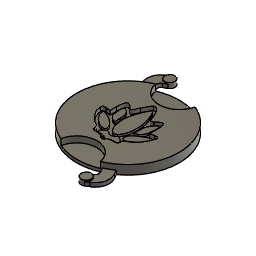
Deckbox - Key - Fungus (Autodesk Fusion 360 design; units mm, degrees)
Autodesk Fusion 360 part; units mm, degrees
sketch "Sketch1" plane through (0, 0, 0) normal (0, 1, 0) x (1, 0, 0)
  circle A0 centre (0, 0) radius 25.4
  line L0 (19.5918, -28.934) -> (-15.2617, 31.434)
  line L1 (-19.5918, 28.934) -> (15.2617, -31.434)
  line L2 (0, -25.4) -> (0, 25.4) construction
  line L3 (0, 0) -> (25.4, 0) construction
  line L4 (-19.5918, 28.934) -> (-15.2617, 31.434)
  line L5 (15.2617, -31.434) -> (19.5918, -28.934)
  line L6 (17.4268, -30.184) -> (-17.4268, 30.184) construction
  line L7 (-2.1651, -1.25) -> (2.1651, 1.25) construction
  line L8 (19.5918, -28.934) -> (11.7976, -33.434)
  line L9 (11.7976, -33.434) -> (9.2976, -29.1039)
  line L10 (9.2976, -29.1039) -> (17.0918, -24.6039)
  line L11 (17.0918, -24.6039) -> (19.5918, -28.934)
  circle A1 centre (10.5476, -31.269) radius 2.5
  circle A2 centre (0, 0) radius 35.5
  line L12 (-19.5918, 28.934) -> (-17.0918, 24.6039)
  line L13 (-17.0918, 24.6039) -> (-9.2976, 29.1039)
  line L14 (-9.2976, 29.1039) -> (-11.7976, 33.434)
  line L15 (-11.7976, 33.434) -> (-19.5918, 28.934)
  circle A3 centre (-10.5476, 31.269) radius 2.5
  point P0 (-12.5, 21.6506)
  point P1 (12.5, -21.6506)
  dimension "d1" = 50.8
  dimension "d42" = 5
  dimension "d45" = 5
  dimension "d46" = 71
  dimension "d47" = 60
  dimension "d48" = 4
  dimension "d51" = 5
  constraint coincident A0.centre L3.start
  constraint coincident A0 L2.start
  constraint coincident A0 L2.end
  constraint coincident A0.centre L2
  constraint coincident A0 L3.end
  constraint horizontal L3
  constraint perpendicular L0 L4
  constraint perpendicular L0 L5
  constraint perpendicular L1 L4
  constraint midpoint L5 L6.start
  constraint midpoint L4 L6.end
  constraint perpendicular L4 L6
  constraint midpoint L1 L7.start
  constraint midpoint L0 L7.end
  constraint midpoint L6 A0.centre
  constraint perpendicular L8 L9
  constraint parallel L8 L10
  constraint parallel L9 L11
  constraint perpendicular L0 L8
  constraint midpoint L9 A1.centre
  constraint tangent L10 A1
  constraint concentric A0 A2
  constraint tangent A1 A2
  constraint perpendicular L12 L13
  constraint parallel L12 L14
  constraint parallel L13 L15
  constraint coincident L1 L12.end
  constraint midpoint L14 A3.centre
  constraint tangent L13 A3
  constraint tangent A2 A3
  measures "d1" diameter of A0
  measures "d42" distance of L0 L1
  measures "d45" diameter of A1
  measures "d46" diameter of A2 A0.centre
  measures "d47" angle of L3 L6
  measures "d48" distance of L1 A1.centre
  measures "d51" diameter of A3
extrude "Extrude1" add sketch "Sketch1" along normal blind 4.5 contours A0 L0 | A0 L0 L1 | A0 L1
extrude "Extrude2" add sketch "Sketch1" along normal blind 1.9 contours A0 L0 | A0 L0 L1 | A0 L0 L1 L13 | A0 L0 L1 L10 | A0 L1 | L0 L1 L4 L12 L13 L15 | L0 L13 L15 A3 | L0 L1 L5 L8 L10 L11 | L14 A3 | L14 A3 | L1 L8 L10 A1 | L9 A1 | L9 A1
extrude "Extrude3" add sketch "Sketch1" along normal blind 2.5 contours L14 A3 | L14 A3 | L9 A1 | L9 A1
sketch "Sketch2" plane through (0, 4.5, 0) normal (0, 1, 0) x (-1, 0, 0)
  circle A0 centre (0, 0) radius 25.4
  circle A1 centre (0, -25.4) radius 10
  circle A2 centre (0, 25.4) radius 10
  line L0 (0, -25.4) -> (0, 25.4) construction
  dimension "d18" = 20
  dimension "d19" = 20
  constraint coincident A0 A1.centre
  constraint coincident A0 A2.centre
  constraint coincident A1.centre L0.start
  constraint coincident A2.centre L0.end
  constraint coincident A0.centre L0
  constraint vertical L0
  measures "d18" diameter of A1
  measures "d19" diameter of A2
extrude "Extrude4" cut sketch "Sketch2" against normal blind 3 contours A0 A2 | A0 A1 picked at (-1.832, 22.0709) picked at (1.832, -22.0709)
fillet "Fillet6" radius 2 2 edges at (12.7617, 0.95, 27.1039) (-12.7617, 0.95, -27.1039)
fillet "Fillet7" radius 7 2 edges at (19.5918, 0.95, 28.934) (-19.5918, 0.95, -28.934)
sketch "Sketch4" plane through (0, 4.5, 0) normal (0, 1, 0) x (-1, 0, 0)
  arc A0 (-9.8043, 23.4315) -> (9.8043, 23.4315) centre (0, 25.4) ccw
  arc A1 (-9.8043, 23.4315) -> (-9.8043, -23.4315) centre (0, 0) ccw
  arc A2 (9.8043, -23.4315) -> (-9.8043, -23.4315) centre (0, -25.4) ccw
  arc A3 (9.8043, -23.4315) -> (9.8043, 23.4315) centre (0, 0) ccw
  spline S0 degree 3 poles (0.8971, -13.3881) (1.2668, -13.1528) (2.3293, -11.3261) (3.2581, -9.3287) knots 0 0 0 0 1 1 1 1
  spline S1 degree 3 poles (3.2581, -9.3287) (4.7374, -6.1473) (5.0418, -5.8117) (5.7137, -6.6214) knots 0 0 0 0 1 1 1 1
  spline S2 degree 3 poles (5.7137, -6.6214) (8.3263, -9.7693) (9.7289, -8.853) (9.7424, -3.9899) knots 0 0 0 0 1 1 1 1
  line L0 (9.7424, -3.9899) -> (9.7512, -0.786)
  line L1 (9.7512, -0.786) -> (11.8532, -1.0314)
  spline S3 degree 3 poles (11.8532, -1.0314) (13.8107, -1.2599) (13.6243, -0.8636) (13.5174, 0.1243) knots 0 0 0 0 1 1 1 1
  spline S4 degree 3 poles (13.5174, 0.1243) (13.3689, 2.9805) (12.268, 3.8405) (11.0374, 5.5764) knots 0 0 0 0 1 1 1 1
  spline S5 degree 3 poles (11.0374, 5.5764) (10.3465, 6.5665) (8.995, 7.7022) (8.0341, 8.1002) knots 0 0 0 0 1 1 1 1
  spline S6 degree 3 poles (8.0341, 8.1002) (6.782, 8.6189) (6.287, 9.213) (6.287, 10.1973) knots 0 0 0 0 1 1 1 1
  spline S7 degree 3 poles (6.287, 10.1973) (6.287, 11.4074) (6.0209, 11.5706) (4.0482, 11.5706) knots 0 0 0 0 1 1 1 1
  spline S8 degree 3 poles (4.0482, 11.5706) (2.7625, 11.5706) (1.5034, 11.9394) (1.0907, 12.4367) knots 0 0 0 0 1 1 1 1
  spline S9 degree 3 poles (1.0907, 12.4367) (0.17, 13.546) (-1.0019, 13.546) (-1.4276, 12.4367) knots 0 0 0 0 1 1 1 1
  spline S10 degree 3 poles (-1.4276, 12.4367) (-1.6469, 11.865) (-2.5511, 11.5706) (-4.0875, 11.5706) knots 0 0 0 0 1 1 1 1
  spline S11 degree 3 poles (-4.0875, 11.5706) (-6.1537, 11.5706) (-6.4151, 11.4164) (-6.4151, 10.1973) knots 0 0 0 0 1 1 1 1
  spline S12 degree 3 poles (-6.4151, 10.1973) (-6.4151, 9.2138) (-6.9098, 8.619) (-8.1576, 8.1021) knots 0 0 0 0 1 1 1 1
  spline S13 degree 3 poles (-8.1576, 8.1021) (-10.4862, 7.1376) (-12.5771, 3.7495) (-13.6607, 0.9406) knots 0 0 0 0 1 1 1 1
  spline S14 degree 3 poles (-13.6607, 0.9406) (-13.8851, 0.3589) (-14.3251, -0.374) (-13.8123, -0.9237) knots 0 0 0 0 1 1 1 1
  spline S15 degree 3 poles (-13.8123, -0.9237) (-13.345, -1.4244) (-12.7159, -1.1171) (-12.0357, -1.0377) knots 0 0 0 0 1 1 1 1
  spline S16 degree 2 poles (-12.0357, -1.0377) (-11.3554, -0.9583) (-9.9948, -0.7994) knots 0 0 0 1 1 1
  line L2 (-9.9948, -0.7994) -> (-9.9948, -4.1027)
  spline S17 degree 3 poles (-9.9948, -4.1027) (-9.9948, -8.9023) (-9.098, -9.5181) (-6.0681, -6.7993) knots 0 0 0 0 1 1 1 1
  spline S18 degree 3 poles (-6.0681, -6.7993) (-4.8607, -5.7158) (-4.8505, -5.7227) (-3.868, -8.2954) knots 0 0 0 0 1 1 1 1
  spline S19 degree 3 poles (-3.868, -8.2954) (-2.2598, -12.5062) (-0.5646, -14.318) (0.8971, -13.3881) knots 0 0 0 0 1 1 1 1
  spline S20 degree 3 poles (-1.6629, -9.6476) (-4.5891, -3.3969) (-4.4153, 3.7702) (-1.2686, 6.6179) knots 0 0 0 0 1 1 1 1
  spline S21 degree 3 poles (-1.2686, 6.6179) (1.4874, 9.1122) (4.7282, 1.5659) (3.3721, -4.1881) knots 0 0 0 0 1 1 1 1
  spline S22 degree 3 poles (3.3721, -4.1881) (2.5694, -7.5939) (0.6122, -12.1015) (-0.0641, -12.1015) knots 0 0 0 0 1 1 1 1
  spline S23 degree 3 poles (-0.0641, -12.1015) (-0.3117, -12.1015) (-1.0312, -10.9972) (-1.6629, -9.6476) knots 0 0 0 0 1 1 1 1
  spline S24 degree 3 poles (-8.4772, -1.4372) (-8.2643, -0.3027) (-7.5442, 0.7079) (-6.5157, 1.3155) knots 0 0 0 0 1 1 1 1
  line L3 (-6.5157, 1.3155) -> (-4.8904, 2.2755)
  line L4 (-4.8904, 2.2755) -> (-4.9872, -0.9697)
  spline S25 degree 3 poles (-4.9872, -0.9697) (-5.0709, -3.7725) (-5.5433, -4.2526) (-6.4664, -5.5741) knots 0 0 0 0 1 1 1 1
  spline S26 degree 3 poles (-6.4664, -5.5741) (-6.9431, -6.2565) (-7.7506, -7.3838) (-8.4359, -7.1095) knots 0 0 0 0 1 1 1 1
  spline S27 degree 3 poles (-8.4359, -7.1095) (-9.039, -6.8681) (-8.8245, -5.7713) (-8.8595, -5.0816) knots 0 0 0 0 1 1 1 1
  spline S28 degree 3 poles (-8.8595, -5.0816) (-8.9214, -3.8617) (-8.6621, -2.4232) (-8.4772, -1.4372) knots 0 0 0 0 1 1 1 1
  spline S29 degree 3 poles (5.9967, -5.1713) (5.2952, -4.3961) (4.9196, -2.9968) (4.8579, -0.9284) knots 0 0 0 0 1 1 1 1
  line L5 (4.8579, -0.9284) -> (4.7658, 2.158)
  line L6 (4.7658, 2.158) -> (6.3459, 1.2511)
  spline S30 degree 3 poles (6.3459, 1.2511) (7.9347, 0.3393) (8.5965, -1.4012) (8.5965, -4.6678) knots 0 0 0 0 1 1 1 1
  spline S31 degree 3 poles (8.5965, -4.6678) (8.5965, -6.6296) (7.5073, -6.8405) (5.9967, -5.1713) knots 0 0 0 0 1 1 1 1
  spline S32 degree 3 poles (9.0206, 1.12) (4.477, 3.0676) (1.8811, 8.0927) (5.8262, 7.3036) knots 0 0 0 0 1 1 1 1
  spline S33 degree 3 poles (5.8262, 7.3036) (8.5154, 6.7659) (12.0607, 2.9704) (12.0607, 0.6293) knots 0 0 0 0 1 1 1 1
  spline S34 degree 3 poles (12.0607, 0.6293) (12.0607, -0.1674) (12.0017, -0.1579) (9.0206, 1.12) knots 0 0 0 0 1 1 1 1
  spline S35 degree 3 poles (-12.1888, 0.6293) (-12.1888, 4.0358) (-5.3436, 9.345) (-4.3362, 6.7198) knots 0 0 0 0 1 1 1 1
  spline S36 degree 3 poles (-4.3362, 6.7198) (-3.782, 5.2754) (-5.5829, 3.0651) (-8.5893, 1.5) knots 0 0 0 0 1 1 1 1
  spline S37 degree 3 poles (-8.5893, 1.5) (-11.6774, -0.1076) (-12.1888, -0.2313) (-12.1888, 0.6293) knots 0 0 0 0 1 1 1 1
  spline S38 degree 3 poles (-0.1831, 8.6838) (-0.675, 8.6838) (-1.3929, 8.3037) (-1.7784, 7.8391) knots 0 0 0 0 1 1 1 1
  spline S39 degree 3 poles (-1.7784, 7.8391) (-2.3919, 7.0999) (-2.6529, 7.1081) (-3.8699, 7.9055) knots 0 0 0 0 1 1 1 1
  spline S40 degree 3 poles (-3.8699, 7.9055) (-5.842, 9.1977) (-5.6919, 10.5482) (-3.6005, 10.3288) knots 0 0 0 0 1 1 1 1
  spline S41 degree 3 poles (-3.6005, 10.3288) (-2.6875, 10.233) (-1.5183, 10.5051) (-1.0023, 10.9334) knots 0 0 0 0 1 1 1 1
  spline S42 degree 3 poles (-1.0023, 10.9334) (-0.2151, 11.5867) (0.087, 11.5867) (0.8742, 10.9334) knots 0 0 0 0 1 1 1 1
  spline S43 degree 3 poles (0.8742, 10.9334) (1.3902, 10.5051) (2.5594, 10.233) (3.4724, 10.3288) knots 0 0 0 0 1 1 1 1
  spline S44 degree 3 poles (3.4724, 10.3288) (5.4801, 10.5394) (5.6373, 9.5684) (3.8332, 8.101) knots 0 0 0 0 1 1 1 1
  spline S45 degree 3 poles (3.8332, 8.101) (2.7045, 7.1829) (2.4145, 7.1518) (1.6226, 7.8641) knots 0 0 0 0 1 1 1 1
  spline S46 degree 3 poles (1.6226, 7.8641) (1.1213, 8.3149) (0.3087, 8.6838) (-0.1831, 8.6838) knots 0 0 0 0 1 1 1 1
extrude "Extrude6" cut sketch "Sketch4" against normal blind 2 contours S0 S1 S2 L0 L1 S3 S4 S5 S6 S7 S8 S9 S10 S11 S12 S13 S14 S15 S16 L2 S17 S18 S19
extrude "Extrude7" cut 6 faces at (-5.3232, 4.5, 0.8269) (-8.9631, 4.5, 2.4434) (-0.9549, 4.5, -6.2321) (-2.6434, 4.5, 8.6473) (10.5699, 4.5, 1.3239) (6.2019, 4.5, -1.7337) along direction (0, -1, 0) blind 1
named bodies: "Deckbox - Key - Fungus"
